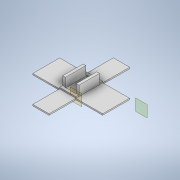
# Autodesk Inventor part: xaxis
Saved by Autodesk Inventor 2021.2 (Build 252289000, 289)
## iProperties
Created: 2021-03-03
Part Number: xaxis
Material: Generic
Document SubType Name: Modeling
Designer: zayda
Density: 1 g/cm^3
Appearance: Default
Author: zayda
Autodesk Inventor part; units mm, degrees
ref_plane "YZ Plane" through (0, 0, 0) normal (1, 0, 0) x (0, 1, 0)
ref_plane "XZ Plane" through (0, 0, 0) normal (0, 1, 0) x (-1, 0, 0)
ref_plane "XY Plane" through (0, 0, 0) normal (0, 0, 1) x (1, 0, 0)
sketch "Sketch1" plane through (0, 0, 0) normal (0, 1, 0) x (-1, 0, 0)
  line L0 (0, 0) -> (-20.5, 0)
  line L1 (-20.5, 0) -> (-20.5, 40.4)
  line L2 (-20.5, 40.4) -> (0, 40.4)
  line L3 (0, 40.4) -> (0, 0)
  line L4 (0, 0) -> (0, -5.08)
  line L5 (0, -5.08) -> (-20.5, -5.08)
  line L6 (-20.5, 0) -> (-20.5, -5.08)
  line L7 (-20.5, -5.08) -> (-25.58, -5.08)
  line L8 (-25.58, -5.08) -> (-25.58, 40.4)
  line L9 (-25.58, 40.4) -> (-25.58, 45.48)
  line L10 (-25.58, 45.48) -> (0, 45.48)
  line L11 (0, 45.48) -> (0, 40.4)
  line L12 (0, -5.08) -> (5.08, -5.08)
  line L13 (5.08, -5.08) -> (5.08, 45.48)
  line L14 (5.08, 45.48) -> (0, 45.48)
  dimension "d0" = 20.5
  dimension "d1" = 40.4
  dimension "d2" = 5.08
  dimension "d3" = 5.08
  dimension "d4" = 5.08
  dimension "d5" = 5.08
  constraints: 30 end point, 7 perpendicular, 4 point on line, 3 parallel, 1 collinear, 1 horizontal, 1 vertical
  measures "d0" distance of L1.end L2.end
  measures "d1" distance of L0.end L1.end
  measures "d2" distance of L0.start L4.end
  measures "d3" distance of L5.end L7.end
  measures "d4" distance of L8.end L9.end
  measures "d5" distance of L4.end L12.end
extrude "Extrusion1" add sketch "Sketch1" along normal blind 25 contours L4 L5 L6 L0 | L3 L11 L14 L13 L12 L4 | L6 L7 L8 L9 L10 L11 L2 L1
sketch "Sketch3" plane through (0, 0, 0) normal (0, -1, 0) x (1, 0, 0)
  line L0 (25.58, 45.48) -> (25.58, -5.08) projected
  line L1 (25.58, -5.08) -> (-5.08, -5.08) projected
  line L2 (25.58, 45.48) -> (-5.08, 45.48)
  line L3 (-5.08, 45.48) -> (-5.08, -5.08)
  line L4 (-5.08, -5.08) -> (25.58, -5.08)
  line L5 (25.58, -5.08) -> (25.58, 45.48)
  point P0 (0, 0)
  constraints: 8 end point, 2 parallel, 1 horizontal, 1 perpendicular
extrude "Extrusion3" add sketch "Sketch3" along normal blind 3.556
sketch "Sketch6" plane through (-5.08, 25, 45.48) normal (0, 0, 1) x (1, 0, 0)
  line L0 (30.66, -28.556) -> (30.66, -28.556) projected
  line L1 (-0.0136, -28.556) -> (30.66, -28.556)
  line L2 (30.66, -28.556) -> (30.66, -26.016)
  line L3 (30.66, -26.016) -> (-0.0136, -26.016)
  line L4 (-0.0136, -26.016) -> (-0.0136, -28.556)
  point P0 (5.08, -25)
  point P1 (-76.2, -28.556)
  point P2 (106.86, -28.556)
  dimension "d17" = 2.54
  constraints: 8 end point, 2 parallel, 1 horizontal, 1 perpendicular, 2 other
  measures "d17" distance of L2.end L1.end
extrude "Extrusion6" [suppressed]
sketch "Sketch7" plane through (25.58, 25, -5.08) normal (0, 0, -1) x (-1, 0, 0)
  line L0 (0, -28.556) -> (0, 0) projected
  line L1 (30.6736, -26.016) -> (0, -26.016) projected
  line L2 (0, -28.556) -> (30.6736, -28.556)
  line L3 (30.6736, -28.556) -> (30.6736, -26.016)
  line L4 (30.6736, -26.016) -> (0, -26.016)
  line L5 (0, -26.016) -> (0, -28.556)
  point P0 (25.58, -25)
  constraints: 8 end point, 2 parallel, 1 horizontal, 1 perpendicular
extrude "Extrusion7" add sketch "Sketch7" along normal blind 50.8
sketch "Sketch9" plane through (0, 25, 0) normal (0, 1, 0) x (1, 0, 0)
  line L0 (-5.0936, 5.08) -> (-5.0936, 55.88) projected
  line L1 (-5.08, -45.48) -> (25.58, -45.48) projected
  line L2 (-5.0936, 5.08) -> (25.58, 5.08)
  line L3 (25.58, 5.08) -> (25.58, -45.48)
  line L4 (25.58, -45.48) -> (-5.0936, -45.48)
  line L5 (-5.0936, -45.48) -> (-5.0936, 5.08)
  point P0 (0, 0)
  constraints: 8 end point, 2 parallel, 1 horizontal, 1 perpendicular
extrude "Extrusion9" cut sketch "Sketch9" against normal blind 7.62
ref_plane "Work Plane1" through (25.58, 1.5293, 45.48) normal (0, 0, 1) x (1, 0, 0)
sketch "Sketch10" plane through (25.58, 1.5293, 45.48) normal (0, 0, 1) x (1, 0, 0)
  line L0 (-30.66, 15.8507) -> (-30.66, 0) projected
  line L1 (-30.66, 15.8507) -> (0, 15.8507)
  line L2 (0, 15.8507) -> (0, 0)
  line L3 (0, 0) -> (-30.66, 0)
  line L4 (-30.66, 0) -> (-30.66, 15.8507)
  point P0 (-25.58, -1.5293)
  constraints: 8 end point, 2 parallel, 1 horizontal, 1 perpendicular
extrude "Extrusion10" cut sketch "Sketch10" against normal blind 6.0325
ref_plane "Work Plane2" through (101.78, 1.5293, -5.08) normal (0, 0, -1) x (-1, 0, 0)
sketch "Sketch11" plane through (101.78, 1.5293, -5.08) normal (0, 0, -1) x (-1, 0, 0)
  line L0 (106.86, 15.8507) -> (106.86, 0) projected
  line L1 (76.2, 0) -> (0, 0) projected
  line L2 (106.86, 15.8507) -> (76.2, 15.8507)
  line L3 (76.2, 15.8507) -> (76.2, 0)
  line L4 (76.2, 0) -> (106.86, 0)
  line L5 (106.86, 0) -> (106.86, 15.8507)
  point P0 (101.78, -1.5293)
  constraints: 8 end point, 2 parallel, 1 horizontal, 1 perpendicular
extrude "Extrusion11" cut sketch "Sketch11" against normal blind 6.0325
sketch "Sketch12" plane through (25.58, 25, -55.88) normal (0, 0, -1) x (-1, 0, 0)
  line L0 (30.6736, -26.016) -> (0, -26.016) projected
  line L1 (0, -26.016) -> (30.6736, -26.016)
  line L2 (30.6736, -26.016) -> (30.6736, -28.556)
  line L3 (30.6736, -28.556) -> (0, -28.556)
  line L4 (0, -28.556) -> (0, -26.016)
  point P0 (25.58, -25)
  constraints: 8 end point, 2 parallel, 1 horizontal, 1 perpendicular
extrude "Extrusion12" cut sketch "Sketch12" against normal blind 50.4825
sketch "Sketch13" plane through (-5.08, -3.556, -5.08) normal (-1, 0, 0) x (0, 0, 1)
  line L0 (0, 0) -> (0, 2.54) projected
  line L1 (50.56, 0) -> (50.56, 5.0853) projected
  line L2 (0, 0) -> (50.56, 0)
  line L3 (50.56, 0) -> (50.56, 2.54)
  line L4 (50.56, 2.54) -> (0, 2.54)
  line L5 (0, 2.54) -> (0, 0)
  point P0 (5.08, 3.556)
  dimension "d32" = 2.54
  constraints: 8 end point, 2 parallel, 1 horizontal, 1 perpendicular, 1 point on line
  measures "d32" distance of L3.end L2.end
extrude "Extrusion13" add sketch "Sketch13" along normal blind 50.4825
sketch "Sketch14" plane through (25.58, 25, -5.3975) normal (0, 0, -1) x (-1, 0, 0)
  line L0 (30.6736, -28.556) -> (0, -28.556) projected
  line L1 (30.6736, -26.016) -> (30.6736, -28.556) projected
  line L2 (0, -28.556) -> (30.6736, -28.556)
  line L3 (30.6736, -28.556) -> (30.6736, -26.016)
  line L4 (30.6736, -26.016) -> (0, -26.016)
  line L5 (0, -26.016) -> (0, -28.556)
  point P0 (25.58, -25)
  constraints: 8 end point, 2 parallel, 1 horizontal, 1 perpendicular
extrude "Extrusion14" add sketch "Sketch14" along normal blind 50.4825
sketch "Sketch15" plane through (25.58, 1.5293, 39.4475) normal (1, 0, 0) x (0, 0, -1)
  line L0 (44.5275, -5.0853) -> (-6.0325, -5.0853) projected
  line L1 (44.5275, -2.5453) -> (-6.0325, -2.5453) projected
  line L2 (-0.0357, -5.0853) -> (44.5275, -5.0853)
  line L3 (44.5275, -5.0853) -> (44.5275, -2.5453)
  line L4 (44.5275, -2.5453) -> (-0.0357, -2.5453)
  line L5 (-0.0357, -2.5453) -> (-0.0357, -5.0853)
  line L6 (-6.0325, -2.5453) -> (-6.0325, -5.0853)
  arc A0 (-4.8702, -5.4467) -> (-6.0325, -5.0853) centre (-6.0325, -7.1351) ccw
  point P0 (39.4475, -1.5293)
  constraints: 10 end point, 2 parallel, 2 perpendicular, 2 point on circle, 1 centre point, 1 horizontal, 1 point on line, 1 tangent
extrude "Extrusion15" add sketch "Sketch15" along normal blind 50.4825
sketch "Sketch16" plane through (-5.08, 1.5293, 45.48) normal (0, 0, 1) x (1, 0, 0)
  line L0 (-0.0136, -5.0853) -> (-0.0136, -2.5453) projected
  line L1 (-0.0136, -2.5453) -> (30.66, -2.5453)
  line L2 (30.66, -2.5453) -> (30.66, -5.1599)
  line L3 (30.66, -5.1599) -> (-0.0136, -5.1599)
  line L4 (-0.0136, -5.1599) -> (-0.0136, -2.5453)
  point P0 (5.08, -1.5293)
  constraints: 8 end point, 2 parallel, 1 horizontal, 1 perpendicular
extrude "Extrusion16" add sketch "Sketch16" along normal blind 50.4825
body "Solid1"
